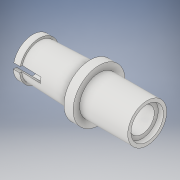
# Autodesk Inventor part: AHHHHHHHHHHHHHHHHHHH
Saved by Autodesk Inventor 2017 (Build 210142000, 142)
## iProperties
Created: 2020-02-20
Part Number: AHHHHHHHHHHHHHHHHHHH
Material: ABS Plastic
Document SubType Name: Modeling
Designer: 10023429
Density: 1.06 g/cm^3
Appearance: Smooth - White
Author: 10023429
Autodesk Inventor part; units mm, degrees
ref_plane "YZ Plane" through (0, 0, 0) normal (1, 0, 0) x (0, 1, 0)
ref_plane "XZ Plane" through (0, 0, 0) normal (0, 1, 0) x (-1, 0, 0)
sketch "Sketch1" plane through (0, 0, 0) normal (0, 0, 1) x (1, 0, 0)
  line L0 (-8.8366, -0.0112) -> (13.5154, -0.0112) construction
  line L1 (-8.8366, -0.6462) -> (-2.4866, -0.6462)
  line L2 (-2.4866, -0.6462) -> (-2.4866, -1.4082)
  line L3 (-2.4866, -1.4082) -> (2.3394, -1.4082)
  line L4 (-8.8366, 1.2588) -> (13.5154, 1.2588) construction
  line L5 (-8.8366, -8.9012) -> (-7.5666, -8.9012) construction
  line L6 (2.3394, -1.4082) -> (2.3394, -3.8212)
  line L7 (4.1174, -1.4082) -> (4.1174, -3.8212)
  line L8 (4.1174, -1.4082) -> (12.4994, -1.4082)
  line L9 (12.4994, -1.4082) -> (12.4994, -0.6462)
  line L10 (12.4994, -0.6462) -> (13.5154, -0.6462)
  line L11 (13.5154, -0.6462) -> (13.5154, -0.0112)
  line L12 (-8.8366, -0.6462) -> (-8.8366, -0.0112)
  line L13 (-8.8366, -0.0112) -> (-7.5666, -0.0112)
  line L14 (-7.5666, -0.0112) -> (-7.5666, -0.3922)
  line L15 (-7.5666, -0.3922) -> (2.3394, -0.0112)
  line L16 (2.3394, -0.0112) -> (2.3394, 1.2588)
  line L17 (2.3394, 1.2588) -> (4.1174, 1.2588)
  line L18 (4.1174, -0.0112) -> (4.1174, 1.2588)
  line L19 (4.1174, -0.0112) -> (13.5154, -0.0112)
  line L20 (-8.8366, -3.8212) -> (15.1492, -3.8212) construction
  line L21 (4.1174, -7.6312) -> (4.1174, -7.6996)
  line L22 (2.3394, -3.8212) -> (4.1174, -3.8212)
  point P0 (0, 0)
  dimension "d0" = 22.352
  dimension "d4" = 0.635
  dimension "d7" = 0.762
  dimension "d11" = 1.27
  dimension "d15" = 8.382
  dimension "d17" = 0.762
  dimension "d18" = 1.27
  dimension "d19" = 0.381
  dimension "d21" = 90
  dimension "d22" = 1.016
  dimension "d23" = 9.398
  dimension "d24" = 9.398
  dimension "d25" = 11.176
  dimension "d26" = 16.002
  dimension "d27" = 1.905
  dimension "d28" = 3.175
  dimension "d29" = 8.255
  dimension "d30" = 13.5154
  dimension "d31" = 0.6462
  dimension "d32" = 1.6337
  dimension "d33" = 0
  dimension "d34" = 6.985
  dimension "d35" = 7.0534
  dimension "d36" = 22.352
  dimension "d37" = 22.352
  constraints: 46 end point, 8 horizontal, 6 point on line, 5 vertical, 4 perpendicular, 3 parallel, 2 midpoint
  measures "d0" distance of L0.start L0.end
  measures "d4" distance between parallel lines of L0 L1
  measures "d7" distance of L1.end L2.end
  measures "d11" distance between parallel lines of L0 L4
  measures "d15" distance of L7.start L8.end
  measures "d17" distance of L8.end L9.end
  measures "d18" distance of L0.start L13.end
  measures "d19" distance of L13.end L14.end
  measures "d21" angle of L10 L16
  measures "d22" distance between parallel lines of L9 L11
  measures "d23" distance between parallel lines of L11 L18
  measures "d24" distance between parallel lines of L21 L11
  measures "d25" distance between parallel lines of L11 L6
  measures "d26" distance between parallel lines of L11 L2
  measures "d27" distance between parallel lines of L17 L10
  measures "d28" distance between parallel lines of L10 L22
  measures "d29" distance between parallel lines of L5 L10
  measures "d30" distance from line of point (0, 0) L11
  measures "d31" distance from line of point (0, 0) L10
  measures "d32" distance from line of L20.end L11
  measures "d33" distance from line of L4.end L11
  measures "d34" distance from line of L21.start L10
  measures "d35" distance from line of L21.end L10
  measures "d36" distance from line of L20.start L11
  measures "d37" distance from line of L5.start L11
revolve "Revolution1" add sketch "Sketch1" angle 360 about axis through (-8.8366, -3.8212, 0) along (1, 0, 0)
ref_plane "Work Plane1" through (-8.2016, -3.8212, 3.81) normal (0, 0, 1) x (1, 0, 0)
sketch "Sketch2" plane through (-8.2016, -3.8212, 3.81) normal (0, 0, 1) x (1, 0, 0)
  line L0 (-0.635, -3.81) -> (-0.635, 3.81) projected
  line L1 (-0.635, 0.8672) -> (4.445, 0.8672)
  line L2 (4.445, 0.8672) -> (4.445, -0.1488)
  line L3 (4.445, -0.1488) -> (-0.635, -0.1488)
  point P0 (8.2016, 3.8212)
  dimension "d44" = 5.08
  dimension "d45" = 1.016
  dimension "d46" = 2.9541
  constraints: 6 end point, 2 perpendicular, 2 point on line, 1 vertical
  measures "d44" distance of L1.start L1.end
  measures "d45" distance of L1.end L2.end
  measures "d46" distance from line of point (8.202, 3.821) L1
extrude "Extrusion1" cut sketch "Sketch2" against normal through all
body "Solid1"
